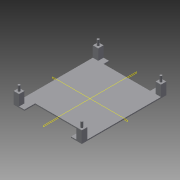
# Autodesk Inventor part: boardtable2
Saved by Autodesk Inventor 2015 SP2 (Build 190223200, 223)
## iProperties
Created: 2016-02-10
Part Number: boardtable2
Material: Generic
Document SubType Name: Modeling
Designer: mca20
Density: 1 g/cm^3
Appearance: Default
Author: mca20
Autodesk Inventor part; units mm, degrees
ref_plane "YZ Plane" through (0, 0, 0) normal (1, 0, 0) x (0, 1, 0)
ref_plane "XZ Plane" through (0, 0, 0) normal (0, 1, 0) x (-1, 0, 0)
ref_plane "XY Plane" through (0, 0, 0) normal (0, 0, 1) x (1, 0, 0)
sketch "Sketch1" plane through (0, 0, 0) normal (0, 1, 0) x (-1, 0, 0)
  line L0 (0, 0) -> (53.34, 0)
  line L1 (53.34, 0) -> (53.34, -68.58)
  line L2 (53.34, -68.58) -> (0, -68.58)
  line L3 (0, -68.58) -> (0, 0)
  line L4 (53.34, -66) -> (0, -66) construction
  circle A0 centre (7.62, -66) radius 1.5
  circle A1 centre (35.56, -66) radius 1.5
  circle A2 centre (2.5, -14) radius 1.5
  line L5 (-5, -73.58) -> (58.34, -73.58)
  line L6 (58.34, -73.58) -> (58.34, 5)
  line L7 (58.34, 5) -> (-5, 5)
  line L8 (-5, 5) -> (-5, -73.58)
  dimension "d0" = 68.58
  dimension "d1" = 53.34
  dimension "d2" = 2.58
  dimension "d3" = 3
  dimension "d4" = 7.62
  dimension "d5" = 3
  dimension "d6" = 35.56
  dimension "d8" = 3
  dimension "d9" = 14
  dimension "d10" = 2.5
  dimension "d46" = 5
  constraints: 18 end point, 4 parallel, 4 point on line, 3 centre point, 3 perpendicular, 1 horizontal, 3 other
  measures "d0" distance between parallel lines of L2 L0
  measures "d1" distance between parallel lines of L3 L1
  measures "d2" distance between parallel lines of L2 L4
  measures "d3" diameter of A0
  measures "d4" distance from line of L3 A0.centre
  measures "d5" diameter of A1
  measures "d6" distance from line of L3 A1.centre
  measures "d8" diameter of A2
  measures "d9" distance from line of L0 A2.centre
  measures "d10" distance from line of L3 A2.centre
  measures "d46" distance between parallel lines of L2 L5
extrude "Extrusion4" add sketch "Sketch1" along normal blind 1 contours L0 L1 L2 L3 | A0 | A1 | A2 | L8 L7 L6 L5
sketch "Sketch5" plane through (0, 1, 0) normal (0, 1, 0) x (1, 0, 0)
  line L0 (5, -5) -> (0, -5)
  line L1 (0, -5) -> (0, 0)
  line L2 (0, 0) -> (5, 0)
  line L3 (5, 0) -> (5, -5)
  dimension "d49" = 5
  dimension "d50" = 5
  constraints: 8 end point, 2 parallel, 1 horizontal, 1 perpendicular
  measures "d49" distance of L1.end L2.end
  measures "d50" distance of L0.end L1.end
extrude "Extrusion5" add sketch "Sketch5" along normal blind 10
ref_plane "Work Plane2" through (-26.67, 0, 5) normal (1, 0, 0) x (0, 0, -1)
mirror "Mirror2" about plane through (-26.67, 0, 5) normal (1, 0, 0) of "Extrusion5"
ref_plane "Work Plane3" through (-58.34, 0, -34.29) normal (0, 0, 1) x (1, 0, 0)
mirror "Mirror3" about plane through (-58.34, 0, -34.29) normal (0, 0, 1) of "Extrusion5", "Mirror2"
sketch "Sketch7" plane through (0, 11, 0) normal (0, 1, 0) x (1, 0, 0)
  line L0 (0, 0) -> (0, -5) projected
  line L1 (0, -5) -> (5, -5) projected
  line L2 (5, -5) -> (5, 0) projected
  line L3 (5, 0) -> (0, 0) projected
  circle A0 centre (2.5, -2.5) radius 0.995
  dimension "d53" = 5
  dimension "d54" = 1.99
  constraints: 1 centre point
  measures "d53" distance between parallel lines of L1 L3
  measures "d54" diameter of A0
extrude "Extrusion8" add sketch "Sketch7" along normal blind 5 contours A0
mirror "Mirror10" about plane through (-26.67, 0, 5) normal (1, 0, 0) of "Extrusion8"
mirror "Mirror11" about plane through (-58.34, 0, -34.29) normal (0, 0, 1) of "Extrusion8", "Mirror10"
sketch "Sketch8" plane through (0, 1, 0) normal (0, 1, 0) x (1, 0, 0)
  line L0 (-53.34, 73.58) -> (-53.34, 68.58) projected
  line L1 (-53.34, 68.58) -> (-58.34, 68.58) projected
  line L2 (-58.34, 68.58) -> (-58.34, 0) projected
  line L3 (-58.34, 0) -> (-53.34, 0) projected
  line L4 (-53.34, 0) -> (-53.34, -5) projected
  line L5 (-53.34, -5) -> (0, -5) projected
  line L6 (0, -5) -> (0, 0) projected
  line L7 (0, 0) -> (5, 0) projected
  line L8 (5, 0) -> (5, 68.58) projected
  line L9 (5, 68.58) -> (0, 68.58) projected
  line L10 (0, 68.58) -> (0, 73.58) projected
  line L11 (0, 73.58) -> (-53.34, 73.58) projected
  line L12 (-58.34, -5) -> (5, -5) projected
  line L13 (-48.34, 5) -> (-5, 5)
  line L14 (-5, 5) -> (-5, -5)
  line L15 (-5, -5) -> (-48.34, -5)
  line L16 (-48.34, -5) -> (-48.34, 5)
  line L17 (5, -5) -> (5, 73.58) projected
  line L18 (5, 73.58) -> (-58.34, 73.58) projected
  line L19 (-48.34, 73.58) -> (-5, 73.58)
  line L20 (-5, 73.58) -> (-5, 68.58)
  line L21 (-5, 68.58) -> (-48.34, 68.58)
  line L22 (-48.34, 68.58) -> (-48.34, 73.58)
  dimension "d64" = 53.34
  dimension "d65" = 43.34
  dimension "d66" = 5
  dimension "d69" = 78.58
  dimension "d72" = 10
  dimension "d73" = 5
  dimension "d74" = 5
  constraints: 16 end point, 4 parallel, 2 horizontal, 2 perpendicular, 2 point on line
  measures "d64" distance between parallel lines of L6 L4
  measures "d65" distance between parallel lines of L14 L16
  measures "d66" distance between parallel lines of L4 L16
  measures "d69" distance between parallel lines of L12 L11
  measures "d72" distance between parallel lines of L15 L13
  measures "d73" distance of L19.end L20.end
  measures "d74" distance between parallel lines of L0 L22
extrude "Extrusion9" cut sketch "Sketch8" against normal blind 1 contours L11 L20 L21 L22 | L16 L13 L14 L5
body "Solid2"
body "Solid3"
